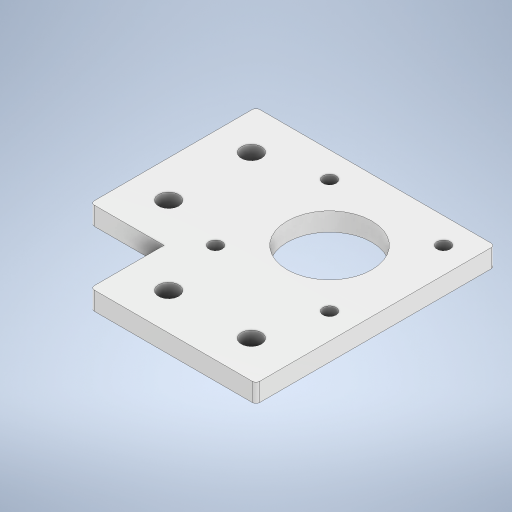
# Autodesk Inventor part: NEMA17 Stepper CornerMount
Saved by Autodesk Inventor 2023 (Build 270158000, 158)
## iProperties
Created: 2023-04-11
Part Number: NEMA17 Stepper CornerMount
Material: PC/ABS Plastic
Document SubType Name: Modeling
Designer: ethan
Density: 0.357273 g/cm^3
Appearance: Smooth - White
Author: ethan
Autodesk Inventor part; units mm, degrees
ref_plane "YZ Plane" through (0, 0, 0) normal (1, 0, 0) x (0, 1, 0)
ref_plane "XZ Plane" through (0, 0, 0) normal (0, 1, 0) x (-1, 0, 0)
ref_plane "XY Plane" through (0, 0, 0) normal (0, 0, 1) x (1, 0, 0)
sketch "Sketch1" plane through (0, 0, 0) normal (0, 1, 0) x (-1, 0, 0)
  line L0 (0, 0) -> (-31, 0) construction
  line L1 (-31, 0) -> (-31, -31) construction
  line L2 (-31, -31) -> (0, -31) construction
  line L3 (0, -31) -> (0, 0) construction
  circle A0 centre (0, 0) radius 1.8
  circle A1 centre (0, -31) radius 1.8
  circle A2 centre (-31, -31) radius 1.8
  circle A3 centre (-31, 0) radius 1.8
  line L4 (-38, 7) -> (-38, -38)
  line L5 (-38, -38) -> (7, -38)
  line L6 (7, -38) -> (27, -38)
  line L7 (27, -38) -> (27, 7)
  line L8 (27, 7) -> (7, 7)
  line L9 (-38, 7) -> (-38, 27)
  line L10 (-38, 27) -> (7, 27)
  line L11 (7, 27) -> (7, 7)
  line L12 (7, 7) -> (-38, -38) construction
  line L13 (-38, 7) -> (7, -38) construction
  line L14 (17, 7) -> (17, -15.5) construction
  line L15 (7, 17) -> (-15.5, 17) construction
  line L16 (-15.5, 27) -> (-15.5, 17) construction
  line L17 (-15.5, 17) -> (-38, 17) construction
  line L18 (27, -15.5) -> (17, -15.5) construction
  line L19 (17, -15.5) -> (17, -38) construction
  circle A4 centre (17, -4.25) radius 2.75
  circle A5 centre (17, -26.75) radius 2.75
  circle A6 centre (-26.75, 17) radius 2.75
  circle A7 centre (-4.25, 17) radius 2.75
  circle A8 centre (-15.5, -15.5) radius 11.5
  dimension "d0" = 31
  dimension "d1" = 31
  dimension "d2" = 3.6
  dimension "d3" = 3.6
  dimension "d4" = 3.6
  dimension "d5" = 3.6
  dimension "d6" = 45
  dimension "d7" = 45
  dimension "d8" = 20
  dimension "d9" = 20
  dimension "d10" = 5.5
  dimension "d11" = 5.5
  dimension "d12" = 5.5
  dimension "d13" = 5.5
  dimension "d17" = 23
  constraints: 40 end point, 12 midpoint, 9 centre point, 9 perpendicular, 4 coincident, 4 parallel, 2 equal length, 2 horizontal, 2 point on line, 1 collinear
  measures "d0" distance of L2.end L1.end
  measures "d1" distance of L1.end L0.end
  measures "d2" diameter of A0
  measures "d3" diameter of A3
  measures "d4" diameter of A2
  measures "d5" diameter of A1
  measures "d6" distance of L5.end L4.end
  measures "d7" distance of L4.start L4.end
  measures "d8" distance of L8.end L7.end
  measures "d9" distance of L4.start L9.end
  measures "d10" diameter of A4
  measures "d11" diameter of A7
  measures "d12" diameter of A5
  measures "d13" diameter of A6
  measures "d17" diameter of A8
extrude "Extrusion1" add sketch "Sketch1" along normal blind 5
fillet "Fillet1" radius 1 5 edges at (-27, 2.5, 7) (-7, 2.5, 27) (38, 2.5, 27) (38, 2.5, -38) (-27, 2.5, -38)
equation "\"d3\" = d2"
equation "\"d4\" = d2"
equation "\"d5\" = d2"
equation "\"d11\" = d10"
equation "\"d12\" = d10"
equation "\"d13\" = d10"
body "Solid1"
